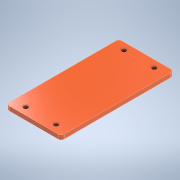
# Autodesk Inventor part: LiPo cover
Saved by Autodesk Inventor 2021 (Build 250183000, 183)
## iProperties
Created: 2020-09-04
Part Number: LiPo cover
Material: Generic
Document SubType Name: Modeling
Designer: jgray
Density: 1 g/cm^3
Appearance: Default
Author: jgray
Autodesk Inventor part; units mm, degrees
ref_plane "YZ Plane" through (0, 0, 0) normal (1, 0, 0) x (0, 1, 0)
ref_plane "XZ Plane" through (0, 0, 0) normal (0, 1, 0) x (-1, 0, 0)
ref_plane "XY Plane" through (0, 0, 0) normal (0, 0, 1) x (1, 0, 0)
sketch "Sketch1" plane through (0, 0, 0) normal (0, 1, 0) x (-1, 0, 0)
  line L0 (-43.5, 202.3853) -> (-0.5, 202.3853) construction
  line L1 (-0.5, 202.3853) -> (-0.5, 140.3853) construction
  line L2 (-0.5, 140.3853) -> (-43.5, 140.3853) construction
  line L3 (-43.5, 140.3853) -> (-43.5, 202.3853) construction
  line L4 (0, 112) -> (0, 260) construction
  line L5 (2.5, 205.3853) -> (-46.5, 205.3853) construction
  line L6 (-46.5, 205.3853) -> (-46.5, 137.3853) construction
  line L7 (-46.5, 137.3853) -> (2.5, 137.3853) construction
  line L8 (2.5, 137.3853) -> (2.5, 205.3853) construction
  line L9 (21.9355, 171.3853) -> (-82.4794, 171.3853) construction
  line L10 (-22, 245.5328) -> (-22, 103.5673) construction
  line L11 (-51.5, 132.3853) -> (7.5, 132.3853)
  line L12 (7.5, 132.3853) -> (7.5, 210.3853)
  line L13 (7.5, 210.3853) -> (-51.5, 210.3853)
  line L14 (-51.5, 210.3853) -> (-51.5, 132.3853)
  line L15 (-51.5, 132.3853) -> (7.5, 210.3853) construction
  line L16 (7.5, 132.3853) -> (-51.5, 210.3853) construction
  point P0 (0, 0)
  point P1 (0, 0)
  point P2 (-13.5, 205.3853)
  point P3 (-34.5, 205.3853)
  point P4 (-46.5, 183.3853)
  point P5 (-46.5, 159.3853)
  point P6 (-34.5, 137.3853)
  point P7 (-13.5, 137.3853)
  point P8 (2.5, 171.3853)
  point P9 (-22, 137.3853)
  point P10 (-22, 171.3853)
  point P11 (0, 132.3853)
  point P12 (0, 210.3853)
  point P13 (-13.5, 205.3853)
  point P14 (-34.5, 205.3853)
  point P15 (-46.5, 183.3853)
  point P16 (-46.5, 159.3853)
  point P17 (-34.5, 137.3853)
  point P18 (-13.5, 137.3853)
  point P19 (2.5, 183.3853)
  point P20 (2.5, 159.3853)
  dimension "d0" = 43
  dimension "d1" = 62
  dimension "d2" = 0.5
  dimension "d3" = 3
  dimension "d4" = 12
  dimension "d5" = 21
  dimension "d6" = 21
  dimension "d7" = 12
  dimension "d8" = 22
  dimension "d9" = 22
  dimension "d10" = 5
  dimension "d11" = 5
  dimension "d28" = 22
  dimension "d29" = 22
  constraints: 34 end point, 16 point on line, 6 coincident, 6 parallel, 4 midpoint, 3 horizontal, 3 perpendicular, 1 vertical, 3 other
  measures "d0" distance of L1.end L2.end
  measures "d1" distance of L0.end L1.end
  measures "d2" distance between parallel lines of L4 L1
  measures "d3" distance between parallel lines of L0 L5
  measures "d4" distance from line of point (-34.5, 205.385) L6
  measures "d5" distance of point (-13.5, 205.385) point (-34.5, 205.385)
  measures "d6" distance of point (-34.5, 137.385) point (-13.5, 137.385)
  measures "d7" distance of point (-34.5, 137.385) L6.end
  measures "d8" distance from line of point (-46.5, 183.385) L5
  measures "d9" distance from line of L7 point (-46.5, 159.385)
  measures "d10" distance between parallel lines of L14 L6
  measures "d11" distance between parallel lines of L11 L7
  measures "d28" distance of point (2.5, 183.385) L5.start
  measures "d29" distance from line of L7 point (2.5, 159.385)
extrude "Extrusion1" add sketch "Sketch1" against normal blind 3
hole "Hole1" at (34.5, 0, 137.3853) at (13.5, 0, 137.3853) at (46.5, 0, 159.3853) at (46.5, 0, 183.3853) at (34.5, 0, 205.3853) at (-2.5, 0, 159.3853) at (-2.5, 0, 183.3853) at (13.5, 0, 205.3853) direction (0, -1, 0) diameter 3.2 end through all
fillet "Fillet1" radius 2 4 edges at (-7.5, -1.5, 210.3853) (51.5, -1.5, 210.3853) (51.5, -1.5, 132.3853) (-7.5, -1.5, 132.3853)
sketch "Sketch2" plane through (0, 0, 0) normal (0, 1, 0) x (1, 0, 0)
  line L0 (49.5, -132.3853) -> (-5.5, -132.3853) projected
  line L1 (-5.5, -210.3853) -> (49.5, -210.3853) projected
  line L2 (5, -132.3853) -> (43, -132.3853)
  line L3 (43, -132.3853) -> (43, -210.3853)
  line L4 (43, -210.3853) -> (5, -210.3853)
  line L5 (5, -210.3853) -> (5, -132.3853)
  arc A0 (-5.5, -132.3853) -> (-7.5, -134.3853) centre (-5.5, -134.3853) ccw projected
  line L6 (-7.5, -134.3853) -> (-7.5, -208.3853) projected
  arc A1 (-7.5, -208.3853) -> (-5.5, -210.3853) centre (-5.5, -208.3853) ccw projected
  line L7 (-5.5, -210.3853) -> (49.5, -210.3853) projected
  arc A2 (49.5, -210.3853) -> (51.5, -208.3853) centre (49.5, -208.3853) ccw projected
  line L8 (51.5, -208.3853) -> (51.5, -134.3853) projected
  arc A3 (51.5, -134.3853) -> (49.5, -132.3853) centre (49.5, -134.3853) ccw projected
  line L9 (49.5, -132.3853) -> (-5.5, -132.3853) projected
  circle A4 centre (-2.5, -183.3853) radius 1.6 projected
  circle A5 centre (34.5, -205.3853) radius 1.6 projected
  circle A6 centre (46.5, -159.3853) radius 1.6 projected
  circle A7 centre (34.5, -137.3853) radius 1.6 projected
  circle A8 centre (13.5, -137.3853) radius 1.6 projected
  circle A9 centre (46.5, -183.3853) radius 1.6 projected
  circle A10 centre (-2.5, -159.3853) radius 1.6 projected
  circle A11 centre (13.5, -205.3853) radius 1.6 projected
  line L10 (24, -128.4136) -> (24, -225.5788) construction
  point P0 (0, 0)
  point P1 (24, -132.3853)
  dimension "d31" = 38
  dimension "d32" = 10.5
  dimension "d34" = 21
  constraints: 10 end point, 3 point on line, 2 parallel, 1 horizontal, 1 midpoint, 1 perpendicular, 1 vertical
  measures "d31" distance between parallel lines of L3 L5
  measures "d32" distance from line of A7.centre L10
  measures "d34" distance of A7.centre A8.centre
extrude "Extrusion2" cut sketch "Sketch2" against normal through all contours A3 L8 A2 L1 L3 L0 | L5 L1 A1 L6 A0 L0
fillet "Fillet2" radius 2 4 edges at (5, -1.5, 210.3853) (43, -1.5, 210.3853) (43, -1.5, 132.3853) (5, -1.5, 132.3853)
equation "\"d32\" = 0.5 * d34"
body "Solid1"
